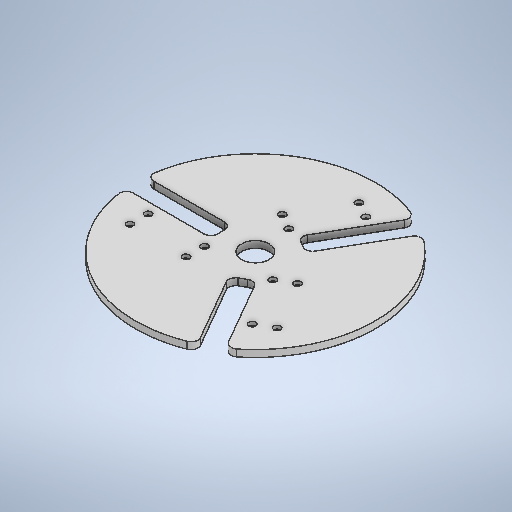
# Autodesk Inventor part: RT_FRM_V2_MC_004_BottomDynamicsPlate
Saved by Autodesk Inventor 2025.3 (Build 293356000, 356)
## iProperties
Created: 2026-04-28
Part Number: RT_FRM_V2_MC_004_BottomDynamicsPlate
Material: Generic
Document SubType Name: Modeling
Designer: louis
Density: 1 g/cm^3
Appearance: Default
Mass: 556.266 g
Surface Area: 1307.88 cm^2
Volume: 556.266 cm^3
Author: louis
Autodesk Inventor part; units mm, degrees
ref_plane "YZ Plane" through (0, 0, 0) normal (1, 0, 0) x (0, 1, 0)
ref_plane "XZ Plane" through (0, 0, 0) normal (0, 1, 0) x (-1, 0, 0)
ref_plane "XY Plane" through (0, 0, 0) normal (0, 0, 1) x (1, 0, 0)
sketch "Sketch1" plane through (0, 0, 0) normal (0, 1, 0) x (-1, 0, 0)
  line L0 (30, -2.5) -> (140, -2.5)
  line L1 (145, 0) -> (25, 0)
  line L2 (0, 0) -> (25, 0)
  circle A0 centre (0, 0) radius 175
  line L3 (50, 0) -> (103.8137, 0) construction
  line L4 (135, 16.5) -> (35, 16.5)
  line L5 (35, 16.5) -> (35, 66.5)
  line L6 (35, 66.5) -> (135, 66.5)
  line L7 (135, 66.5) -> (135, 16.5)
  line L8 (85, 16.5) -> (85, 0) construction
  line L9 (85, 66.5) -> (85, 16.5) construction
  line L10 (126, 30.5) -> (85, 30.5) construction
  line L11 (126, 30.5) -> (126, 57) construction
  line L12 (174.356, -15) -> (50, -15)
  line L13 (50, -15) -> (50, 15)
  line L14 (50, 15) -> (174.356, 15)
  line L15 (174.356, 15) -> (174.356, -15)
  line L16 (0, 0) -> (0, 175)
  line L17 (160, 15) -> (160, 115)
  line L18 (160, 115) -> (-66.3953, 115)
  line L19 (-66.3953, 115) -> (0, 0)
  circle A1 centre (0, 0) radius 310 construction
  line L20 (-310, -390) -> (-310, -310) construction
  line L21 (-310, -310) -> (-390, -310) construction
  line L22 (-390, -310) -> (-390, -390) construction
  line L23 (-390, -390) -> (-310, -390) construction
  line L24 (-310, -390) -> (-390, -310) construction
  line L25 (-310, -310) -> (-390, -390) construction
  line L26 (-310, 310) -> (-310, 390) construction
  line L27 (-310, 390) -> (-390, 390) construction
  line L28 (-390, 390) -> (-390, 310) construction
  line L29 (-390, 310) -> (-310, 310) construction
  line L30 (-310, 310) -> (-390, 390) construction
  line L31 (-310, 390) -> (-390, 310) construction
  line L32 (390, 310) -> (390, 390) construction
  line L33 (390, 390) -> (310, 390) construction
  line L34 (310, 390) -> (310, 310) construction
  line L35 (310, 310) -> (390, 310) construction
  line L36 (390, 310) -> (310, 390) construction
  line L37 (390, 390) -> (310, 310) construction
  line L38 (390, -390) -> (390, -310) construction
  line L39 (390, -310) -> (310, -310) construction
  line L40 (310, -310) -> (310, -390) construction
  line L41 (310, -390) -> (390, -390) construction
  line L42 (390, -390) -> (310, -310) construction
  line L43 (390, -310) -> (310, -390) construction
  line L44 (310, -310) -> (310, 310) construction
  line L45 (310, 310) -> (-310, 310) construction
  line L46 (-310, 310) -> (-310, -310) construction
  line L47 (-310, -310) -> (310, -310) construction
  line L48 (-66.3953, 115) -> (-87.5, 151.5544)
  line L49 (160, 15) -> (174.356, 15)
  line L50 (-100.1684, 143.4967) -> (-74.1876, 158.4967)
  line L51 (-74.1876, -158.4967) -> (-100.1684, -143.4967)
  point P0 (44, 30.5)
  point P1 (44, 57)
  point P2 (162.4808, -65)
  point P3 (50, 0)
  point P4 (-74.1876, 158.4967)
  point P5 (-87.178, 150.9967)
  point P6 (160, 70.8872)
  point P7 (131.9091, 115)
  point P8 (0, 115)
  dimension "d0" = 110
  dimension "d2" = 2.5
  dimension "d4" = 85
  dimension "d9" = 350
  dimension "d11" = 19
  dimension "d12" = 50
  dimension "d13" = 100
  dimension "d14" = 26.5
  dimension "d15" = 82
  dimension "d26" = 30
  dimension "d27" = 35
  dimension "d33" = 9.5
  dimension "d40" = 50
  dimension "d46" = 120
  dimension "d47" = 100
  dimension "d48" = 25
  dimension "d74" = 80
  dimension "d75" = 80
  dimension "d78" = 80
  dimension "d79" = 80
  dimension "d80" = 80
  dimension "d81" = 80
  dimension "d82" = 80
  dimension "d83" = 80
  dimension "d86" = 620
  dimension "d97" = 360
  constraints: 104 end point, 14 perpendicular, 12 parallel, 7 vertical, 5 point on circle, 4 horizontal, 4 point on line, 3 coincident, 3 midpoint, 3 tangent, 2 centre point, 2 collinear, 2 symmetric about line, 10 other
  measures "d0" distance of L0.end L0.start
  measures "d2" distance between parallel lines of L0 L1
  measures "d4" distance of L2.start L8.end
  measures "d9" diameter of A0
  measures "d11" distance from line of L0 L4.start
  measures "d12" distance of L6.end L4.start
  measures "d13" distance of L4.start L4.end
  measures "d14" distance of L11.end L10.start
  measures "d15" distance of L10.start point (44, 30.5)
  measures "d26" distance between parallel lines of L14 L12
  measures "d27" distance between parallel lines of L8 L13
  measures "d33" distance from line of L6 L11.end
  measures "d40" distance from line of L12 point (162.481, -65)
  measures "d46" angle of L19 L2
  measures "d47" distance of L17.start L17.end
  measures "d48" distance between parallel lines of L17 L7
  measures "d74" distance of L21.end L22.end
  measures "d75" distance of L22.end L20.start
  measures "d78" distance of L27.end L28.end
  measures "d79" distance of L28.end L26.start
  measures "d80" distance of L33.end L34.end
  measures "d81" distance of L34.end L32.start
  measures "d82" distance of L39.end L40.end
  measures "d83" distance of L40.end L38.start
  measures "d86" distance of L34.end L26.start
extrude "Extrusion1" add sketch "Sketch1" against normal blind 10 contours L1 L2 L16 L18 A0 L17 L14 L13 | L19 L18 L16 | L17 A0 L14 | L18 L48 L50 A0 L16 | L16 A0 L18 | L4 L5 L6 L7
pattern_circular "Circular Pattern2" count 3 over 360 about axis through (0, 0, 0) along (0, -1, 0) of "Extrusion1"
hole "Hole1" at (-126, 0, 30.5) at (-44, 0, 30.5) at (-126, 0, 57) at (-44, 0, 57) direction (0, -1, 0) diameter 5.5 end through all counterbore diameter 10 counterbore depth 5 clearance for "Socket Head Cap Screw" size "M5" standard "Ansi Metric M Profile"
extrude "Extrusion2" cut sketch "Sketch1" against normal blind 10 contours L13 L14 L15 L12
pattern_circular "Circular Pattern1" count 3 over 360 about axis through (0, -10, 0) along (0, 1, 0) of "Hole1", "Extrusion2"
fillet "Fillet1" radius 10 6 edges at (12.0096, -5, 50.8013) (37.9904, -5, -35.8013) (-50, -5, -15) (-50, -5, 15) (37.9904, -5, 35.8013) (12.0096, -5, -50.8013)
sketch "Sketch3" plane through (0, -10, 0) normal (0, -1, 0) x (1, 0, 0)
  arc A0 (74.1876, 158.4967) -> (-174.356, 15) centre (0, 0) ccw projected
  line L0 (0, 0) -> (-392.8558, 0)
  line L1 (0, 0) -> (87.5, 151.5544)
  circle A1 centre (0, 0) radius 20
  arc A2 (100.1684, -143.4967) -> (100.1684, 143.4967) centre (0, 0) ccw projected
  line L2 (-35.75, 35.75) -> (35.75, 35.75) construction
  line L3 (35.75, 35.75) -> (35.75, -35.75) construction
  line L4 (35.75, -35.75) -> (-35.75, -35.75) construction
  line L5 (-35.75, -35.75) -> (-35.75, 35.75) construction
  line L6 (-35.75, 35.75) -> (35.75, -35.75) construction
  line L7 (35.75, 35.75) -> (-35.75, -35.75) construction
  point P0 (141.3901, 103.1204)
  point P1 (100.1684, 143.4967)
  dimension "d99" = 120
  dimension "d100" = 40
  dimension "d101" = 71.5
  dimension "d102" = 71.5
  constraints: 16 end point, 2 horizontal, 2 midpoint, 2 parallel, 1 centre point, 1 coincident, 1 perpendicular, 1 point on circle
  measures "d99" angle of L0 L1
  measures "d100" diameter of A1
  measures "d101" distance of L3.end L4.end
  measures "d102" distance of L2.end L3.end
extrude "Extrusion3" cut sketch "Sketch3" against normal up to surface (10 mm away)
fillet "Fillet2" radius 10 6 edges at (-174.356, -5, 15) (-174.356, -5, -15) (100.1684, -5, -143.4967) (100.1684, -5, 143.4967) (74.1876, -5, 158.4967) (74.1876, -5, -158.4967)
body "Solid1"
